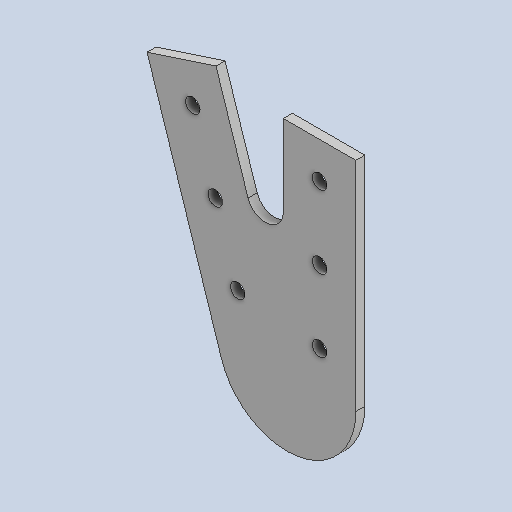
# Autodesk Inventor part: Top_angled_gusset
Saved by Autodesk Inventor 2024 (Build 280153000, 153)
## iProperties
Created: 2023-04-21
Part Number: Top_angled_gusset
Material: Generic
Document SubType Name: Modeling
Designer: legom
Density: 1 g/cm^3
Appearance: Default
Author: legom
Autodesk Inventor part; units mm, degrees
ref_plane "YZ Plane" through (0, 0, 0) normal (1, 0, 0) x (0, 1, 0)
ref_plane "XZ Plane" through (0, 0, 0) normal (0, 1, 0) x (-1, 0, 0)
ref_plane "XY Plane" through (0, 0, 0) normal (0, 0, 1) x (1, 0, 0)
sketch "Sketch1" plane through (0, 0, 0) normal (0, 0, 1) x (1, 0, 0)
  line L0 (0, 0) -> (-25.4, 0)
  line L1 (-25.4, 0) -> (-25.4, 76.2)
  line L2 (-25.4, 76.2) -> (0, 76.2)
  line L3 (0, 76.2) -> (0, 0)
  line L4 (-25.4, 7.874) -> (-49.5487, 0)
  line L5 (-49.5487, 0) -> (-73.1707, 72.4461)
  line L6 (-73.1707, 72.4461) -> (-49.022, 80.3201)
  line L7 (-49.022, 80.3201) -> (-25.4, 7.874)
  circle A0 centre (-24.1487, 0) radius 24.1487
  line L8 (-49.5487, 0) -> (-47.1078, -7.4861)
  dimension "d0" = 25.4
  dimension "d1" = 76.2
  dimension "d3" = 25.4
  dimension "d4" = 7.874
  dimension "d5" = 76.2
  constraints: 18 end point, 4 parallel, 3 tangent, 2 perpendicular, 2 point on circle, 2 point on line, 1 centre point, 1 horizontal
  measures "d0" distance of L1.end L2.end
  measures "d1" distance of L0.end L1.end
  measures "d3" distance of L4.start L4.end
  measures "d4" distance of L0.end L4.start
  measures "d5" distance of L4.end L5.end
extrude "Extrusion1" add sketch "Sketch1" along normal blind 3.175 contours A0 L4 L1 L0 | A0 L1 L2 L3 | L0 L1 A0 | L8 L4 A0 | L4 A0 L7 | L4 L5 L6 L7 A0
fillet "Fillet1" radius 6.35 1 edges at (-25.4, 7.874, 1.5875)
sketch "Sketch2" plane through (0, 0, 3.175) normal (0, 0, 1) x (1, 0, 0)
  line L0 (0, 76.2) -> (-25.4, 76.2) projected
  line L1 (-25.4, 76.2) -> (-25.4, 47.8326) projected
  arc A0 (-37.7872, 45.8641) -> (-25.4, 47.8326) centre (-31.75, 47.8326) ccw projected
  line L2 (-37.7872, 45.8641) -> (-49.022, 80.3201) projected
  line L3 (-49.022, 80.3201) -> (-73.1707, 72.4461) projected
  line L4 (-73.1707, 72.4461) -> (-47.1078, -7.4861) projected
  arc A1 (-47.1078, -7.4861) -> (0, 0) centre (-24.1487, 0) ccw projected
  line L5 (0, 0) -> (0, 76.2) projected
  circle A2 centre (-12.7, 63.5) radius 2.5527
  circle A3 centre (-12.7, 38.1) radius 2.5527
  circle A4 centre (-12.7, 12.7) radius 2.5527
  circle A5 centre (-57.1594, 64.3088) radius 2.5527
  circle A6 centre (-49.2854, 40.1601) radius 2.5527
  circle A7 centre (-41.4114, 16.0114) radius 2.5527
  dimension "d9" = 5.1054
  dimension "d10" = 12.7
  dimension "d11" = 12.7
  dimension "d14" = 25.4
  dimension "d19" = 5.1054
  dimension "d20" = 12.7
  dimension "d21" = 12.7
  dimension "d24" = 25.4
  constraints: 6 centre point, 1 vertical, 9 other
  measures "d9" diameter of A2
  measures "d10" distance from line of L0 A2.centre
  measures "d11" distance from line of L1 A2.centre
  measures "d14" distance of A2.centre A3.centre
  measures "d19" diameter of A5
  measures "d20" distance from line of L4 A5.centre
  measures "d21" distance from line of L3 A5.centre
  measures "d24" distance of A5.centre A6.centre
extrude "Extrusion2" cut sketch "Sketch2" against normal blind 3.175 contours A2 | A3 | A4 | A5 | A6 | A7
body "Solid1"
